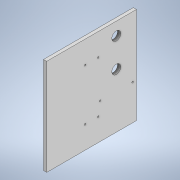
# Autodesk Inventor part: Part_B9
Saved by Autodesk Inventor 2022.6 (Build 266554010, 554A)
## iProperties
Created: 2025-06-02
Part Number: Part_B9
Material: Generic
Document SubType Name: Modeling
Designer: khinm
Density: 1 g/cm^3
Appearance: Default
Author: khinm
Autodesk Inventor part; units mm, degrees
ref_plane "YZ Plane" through (0, 0, 0) normal (1, 0, 0) x (0, 1, 0)
ref_plane "XZ Plane" through (0, 0, 0) normal (0, 1, 0) x (-1, 0, 0)
ref_plane "XY Plane" through (0, 0, 0) normal (0, 0, 1) x (1, 0, 0)
sketch "Sketch1" plane through (0, 0, 0) normal (1, 0, 0) x (0, 1, 0)
  line L0 (75, 70) -> (-75, 70)
  line L1 (-75, 70) -> (-75, -70)
  line L2 (-75, -70) -> (75, -70)
  line L3 (75, -70) -> (75, 70)
  point P0 (0, 0)
  point P1 (75, 0)
  point P2 (0, 70)
  dimension "d0" = 140
  dimension "d1" = 150
  constraints: 8 end point, 2 midpoint, 2 parallel, 1 horizontal, 1 horizontal alignment, 1 perpendicular, 1 vertical alignment
  measures "d0" distance of L2.end L0.start
  measures "d1" distance of L1.end L2.end
extrude "Extrusion1" add sketch "Sketch1" along normal mid plane 5
sketch "Sketch2" plane through (2.5, 0, 0) normal (1, 0, 0) x (0, 0, -1)
  line L0 (70, 75) -> (-70, 75) projected
  line L1 (-10.18, 40) -> (10.18, 40)
  point P0 (0, 0)
  point P1 (0, 40)
  dimension "d4" = 20.36
  dimension "d5" = 35
  constraints: 2 end point, 1 horizontal, 1 horizontal alignment, 1 midpoint, 1 vertical alignment
  measures "d4" distance of L1.end L1.start
  measures "d5" distance from line of L0 L1.start
hole "Hole1" at (2.5, 40, 10.18) at (2.5, 40, -10.18) direction (-1, 0, 0) diameter 2.4 depth 4
pattern_linear "Rectangular Pattern1" count 2 spacing 80 along (0, -1, 0) of "Hole1"
sketch "Sketch3" plane through (2.5, 0, 0) normal (1, 0, 0) x (0, 0, -1)
  circle A0 centre (10.18, -40) radius 1.2 projected
  point P0 (0, 0)
  point P1 (13.0561, -20)
  point P2 (63.8461, -20)
  dimension "d16" = 50.79
  dimension "d19" = 20
  dimension "d20" = 13.0561
  constraints: 1 horizontal alignment
  measures "d16" distance of point (63.846, -20) point (13.056, -20)
  measures "d19" vertical distance of A0.centre point (13.056, -20)
  measures "d20" horizontal distance of point (13.056, -20) point (0, 0)
hole "Hole2" at (2.5, -20, -13.0561) at (2.5, -20, -63.8461) direction (-1, 0, 0) diameter 2.4 depth 4
sketch "Sketch4" plane through (2.5, 0, 0) normal (1, 0, 0) x (0, 0, -1)
  line L0 (70, 75) -> (-70, 75) projected
  circle A0 centre (13.0561, -20) radius 1.2 projected
  circle A1 centre (63.8461, -20) radius 1.2 projected
  line L1 (13.0561, -20) -> (63.8461, -20)
  point P0 (0, 0)
  point P1 (38.4511, 55)
  point P2 (38.4511, -20)
  point P3 (38.4511, 10)
  dimension "d28" = 20
  dimension "d29" = 45
  constraints: 2 end point, 2 vertical alignment, 1 horizontal, 1 midpoint
  measures "d28" distance from line of point (38.451, 55) L0
  measures "d29" distance of point (38.451, 10) point (38.451, 55)
hole "Hole3" at (2.5, 55, -38.4511) at (2.5, 10, -38.4511) direction (-1, 0, 0) diameter 14 depth 5
body "Solid1"
